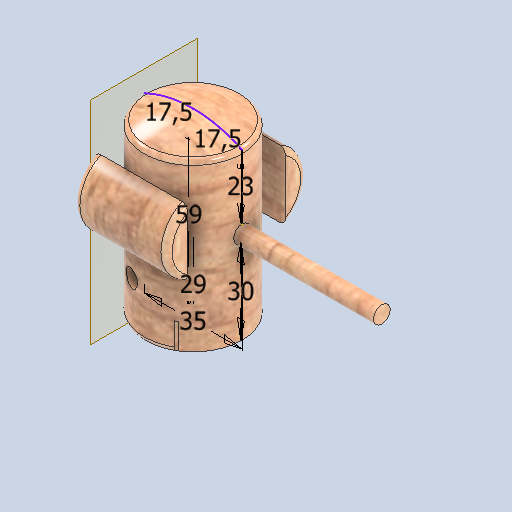
# Autodesk Inventor part: hlava
Saved by Autodesk Inventor 2025.2 (Build 292293000, 293)
## iProperties
Created: 2025-04-28
Part Number: hlava
Material: Wood (Birch)
Document SubType Name: Modeling
Designer: fanda
Density: 0.55 g/cm^3
Appearance: Birch - Natural Polished
Author: fanda
Autodesk Inventor part; units mm, degrees
sketch "Sketch1" plane through (0, 0, 0) normal (0, 0, 1) x (1, 0, 0)
  line L0 (-7.6489, 1.3737) -> (42.3511, 1.3737)
  line L1 (-7.6489, 1.3737) -> (-7.6489, -4.6263)
  line L2 (-7.6489, -4.6263) -> (42.3511, -4.6263)
  line L3 (42.3511, -4.6263) -> (42.3511, 1.3737)
  line L4 (42.3511, -1.6263) -> (-7.6489, -1.6263)
  point P0 (0, 0)
  dimension "d0" = 50
  dimension "d1" = 6
  dimension "d2" = 50
  dimension "d3" = 50
  constraints: 10 end point, 2 horizontal, 2 midpoint, 1 vertical
  measures "d0" distance of L0.start L0.end
  measures "d1" distance of L0.start L1.end
  measures "d2" distance of L1.end L2.end
  measures "d3" distance of L4.start L4.end
revolve "Revolution1" add sketch "Sketch1" angle 360 about axis through (42.3511, -1.6263, 0) along (-1, 0, 0) contours L0 L3 L4 L1
ref_plane "Work Plane3" through (-7.649, 0, 0) normal (1, 0, 0) x (0, 1, 0)
sketch "Sketch2" plane through (0, 0, 0) normal (0, 0, 1) x (1, 0, 0)
  line L0 (-7.6489, 1.3737) -> (-7.6489, -4.6263) projected
  line L1 (-7.6489, 1.3737) -> (-7.6489, 24.3737)
  line L2 (-7.6489, -4.6263) -> (-7.6489, -34.6263)
  line L3 (-7.6489, 24.3737) -> (-25.1489, 24.3737)
  line L4 (-25.1489, 24.3737) -> (-25.1489, -34.6263)
  line L5 (-25.1489, -34.6263) -> (-7.6489, -34.6263)
  arc A0 (-7.6489, 24.3737) -> (-42.6489, 24.3737) centre (-25.1489, -11.595) ccw
  line L6 (-25.1489, 24.3737) -> (-25.1489, 28.405)
  arc A1 (-42.6489, -34.6263) -> (-7.6489, -34.6263) centre (-25.1489, -11.5017) ccw
  line L7 (-25.1489, -34.6263) -> (-25.1489, -40.5017)
  point P0 (0, 0)
  dimension "d7" = 23
  dimension "d8" = 30
  dimension "d9" = 17.5
  dimension "d10" = 59
  dimension "d13" = 17.5
  dimension "d15" = 35
  dimension "d16" = 29
  constraints: 14 end point, 6 point on circle, 2 centre point, 2 vertical, 1 horizontal, 1 perpendicular, 1 point on line
  measures "d7" distance of L0.start L1.end
  measures "d8" distance of L0.end L2.end
  measures "d9" distance of L1.end L3.end
  measures "d10" distance of L3.end L4.end
  measures "d13" distance of L3.end A0.end
  measures "d15" distance of L2.end A1.start
  measures "d16" radius of A1
revolve "Revolution2" add sketch "Sketch2" angle 360 about axis through (-25.1489, 24.3737, 0) along (0, -1, 0)
sketch "Sketch4" plane through (0, 0, 0) normal (0, 0, 1) x (1, 0, 0)
  line L0 (-42.6489, -34.6263) -> (-7.6489, -34.6263) projected
  line L1 (-7.6489, -34.6263) -> (-15.6489, -34.6263)
  arc A0 (-42.6489, -34.6263) -> (-7.6489, -34.6263) centre (-25.1489, -11.5017) ccw projected
  line L2 (-7.6489, -34.6263) -> (-7.6489, -40.5017)
  line L3 (-7.6489, -40.5017) -> (-15.6489, -40.5017)
  line L4 (-15.6489, -40.5017) -> (-15.6489, -25.5017)
  line L5 (-15.6489, -25.5017) -> (-16.6489, -25.5017)
  line L6 (-16.6489, -25.5017) -> (-16.6489, -40.5017)
  line L7 (-16.6489, -40.5017) -> (-15.6489, -40.5017)
  line L8 (-42.6489, -34.6263) -> (-42.6489, -40.5017)
  line L9 (-42.6489, -40.5017) -> (-42.6489, -18.5017)
  line L10 (-42.6489, 24.3737) -> (-42.6489, -34.6263) projected
  line L11 (-42.6489, -18.5017) -> (-30.6489, -18.5017)
  circle A1 centre (-30.6489, -18.5017) radius 3
  line L12 (-42.6489, -40.5017) -> (-42.6489, -28.5017)
  line L13 (-42.6489, -28.5017) -> (-45.6489, -28.5017)
  line L14 (-47.6489, -26.5017) -> (-47.6489, -25.5017)
  line L15 (-47.6489, -25.5017) -> (-42.6489, -25.5017)
  arc A2 (-47.6489, -26.5017) -> (-45.6489, -28.5017) centre (-45.6489, -26.5017) ccw
  point P0 (0, 0)
  point P1 (-47.6489, -28.5017)
  dimension "d19" = 8
  dimension "d23" = 8
  dimension "d24" = 15
  dimension "d25" = 1
  dimension "d27" = 22
  dimension "d28" = 12
  dimension "d29" = 6
  dimension "d32" = 12
  dimension "d33" = 5
  dimension "d34" = 3
  dimension "d35" = 2
  constraints: 28 end point, 7 perpendicular, 7 point on line, 2 centre point, 2 point on circle, 2 tangent, 2 vertical, 1 coincident, 1 horizontal, 1 parallel
  measures "d19" distance of L0.end L1.end
  measures "d23" distance of L2.end L3.end
  measures "d24" distance of L3.end L4.end
  measures "d25" distance of L4.end L5.end
  measures "d27" distance of L8.end L9.end
  measures "d28" distance of L9.end L11.end
  measures "d29" diameter of A1
  measures "d32" distance of L8.end L12.end
  measures "d33" distance of L12.end point (-47.649, -28.502)
  measures "d34" distance of point (-47.649, -28.502) L14.end
  measures "d35" radius of A2
extrude "Extrusion2" cut sketch "Sketch4" along normal mid plane 550 contours L4 A0 L6 L0 | L0 L6 L5 L4 | L4 L7 L6 A0 | A1
revolve "Revolution3" add sketch "Sketch4" angle 360 about axis through (-47.6489, -25.5017, 0) along (1, 0, 0) contours L13 A2 L14 L15 L9
fillet "Fillet1" radius 2 1 edges at (-42.6489, 24.3737, 0)
fillet "Fillet2" radius 2 1 edges at (-42.6489, -34.6263, 0)
ref_plane "Work Plane6" through (0, 0, -17.5) normal (0, 0, 1) x (1, 0, 0)
ref_plane "Work Plane7" through (-25.1489, -5.1263, 17.5) normal (0, 0, 1) x (1, 0, 0)
sketch "Sketch7" plane through (0, 0, -17.5) normal (0, 0, 1) x (1, 0, 0)
  arc A0 (-41.4647, 24.9261) -> (-42.6489, 23.1001) centre (-40.6489, 23.1001) ccw projected
  line L0 (-42.6489, 23.1001) -> (-42.6489, 3.1001)
  line L1 (-42.6489, 3.1001) -> (-25.1489, 3.1001)
  line L2 (-25.1489, 3.1001) -> (-10.6489, 3.1001)
  line L3 (-10.6489, 3.1001) -> (-10.6489, -8.8999)
  line L4 (-10.6489, -8.8999) -> (-43.6489, -8.8999)
  line L5 (-43.6489, -8.8999) -> (-43.6489, 15.1001)
  line L6 (-43.6489, 15.1001) -> (-10.6489, 15.1001)
  line L7 (-10.6489, 15.1001) -> (-10.6489, 3.1001)
  line L8 (-10.6489, 3.1001) -> (-43.6489, 3.1001)
  point P0 (0, 0)
  dimension "d41" = 20
  dimension "d42" = 17.5
  dimension "d43" = 14.5
  dimension "d44" = 12
  dimension "d45" = 33
  dimension "d46" = 24
  dimension "d47" = 33
  constraints: 18 end point, 5 perpendicular, 1 horizontal, 1 midpoint, 1 point on circle, 1 point on line, 1 tangent, 1 vertical
  measures "d41" distance of L0.start L0.end
  measures "d42" distance of L0.end L1.end
  measures "d43" distance of L1.end L2.end
  measures "d44" distance of L2.end L3.end
  measures "d45" distance of L3.end L4.end
  measures "d46" distance of L4.end L5.end
  measures "d47" distance of L5.end L6.end
ref_plane "Work Plane8" through (-42.6489, -5.1263, 0) normal (1, 0, 0) x (0, 0, -1)
sketch "Sketch8" plane through (-42.6489, -5.1263, 0) normal (1, 0, 0) x (0, 0, -1)
  arc A0 (17.5, 28.2264) -> (16.3158, 30.0524) centre (15.5, 28.2264) ccw projected
  line L0 (17.5, 28.2264) -> (17.5, -28.483) projected
  line L1 (17.5, 28.2264) -> (17.5, 20.2264)
  line L2 (17.5, 20.2264) -> (17.5, -3.7736)
  line L3 (17.5, 8.2264) -> (25, 8.2264)
  arc A1 (17.5, -3.7736) -> (17.5, 20.2264) centre (11.65, 8.2264) ccw
  arc A2 (-16.3158, 30.0524) -> (-17.5, 28.2264) centre (-15.5, 28.2264) ccw projected
  line L4 (-17.5, 28.2264) -> (-17.5, 20.2264)
  arc A3 (-16.3158, 30.0524) -> (-17.5, 28.2264) centre (-15.5, 28.2264) ccw projected
  line L5 (-17.5, 20.2264) -> (-17.5, -3.7736)
  line L6 (-17.5, 8.2264) -> (-25, 8.2264)
  arc A4 (-17.5, 20.2264) -> (-17.5, -3.7736) centre (-11.65, 8.2264) ccw
  point P0 (0, 5.1263)
  dimension "d49" = 8
  dimension "d50" = 24
  dimension "d51" = 7.5
  dimension "d54" = 8
  dimension "d55" = 24
  dimension "d56" = 7.5
  constraints: 12 end point, 7 point on circle, 3 point on line, 2 centre point, 2 horizontal, 2 midpoint, 1 tangent, 1 vertical
  measures "d49" distance of L0.start L1.end
  measures "d50" distance of L1.end L2.end
  measures "d51" distance of L3.start L3.end
  measures "d54" distance of L4.start L4.end
  measures "d55" distance of L4.end L5.end
  measures "d56" distance of L6.start L6.end
extrude "Extrusion3" add sketch "Sketch8" along normal blind 33
fillet "Fillet3" radius 2 4 edges at (-42.6489, 3.1001, -25) (-9.6489, 3.1001, -25) (-42.6489, 3.1001, 25) (-9.6489, 3.1001, 25)
